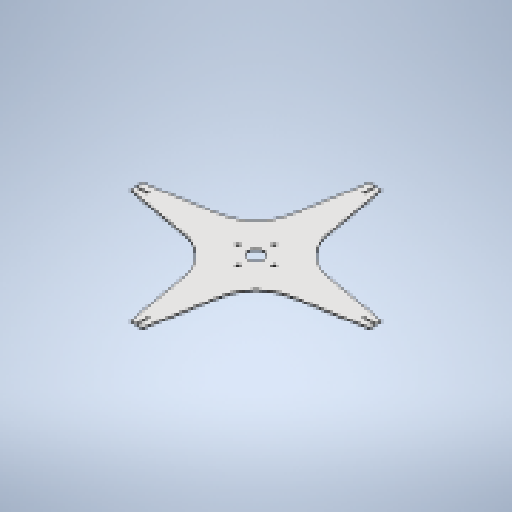
# Autodesk Inventor part: TRM 030 star main
Saved by Autodesk Inventor 2025 (Build 290162010, 162A)
## iProperties
Created: 2024-08-07
Part Number: TRM 030 star main
Material: AISI 304
Document SubType Name: Sheet Metal
Designer: admin
Stock Number: ТРМ 015 левый борт основное
Density: 8.02768 g/cm^3
Flat Pattern Width: 39.95 cm
Flat Pattern Length: 39.95 cm
Flat Pattern Area: 1596 cm^2
Sheet Metal Rule: AISI304 2mm Die16
Sheet Metal Width: 399,500 mm
Sheet Metal Length: 399,500 mm
Sheet Metal Area: 159600,000 mm^2
Appearance: Default
Author: pokla
Autodesk Inventor part; units mm, degrees
ref_plane "YZ Plane" through (0, 0, 0) normal (1, 0, 0) x (0, 1, 0)
ref_plane "XZ Plane" through (0, 0, 0) normal (0, 1, 0) x (-1, 0, 0)
ref_plane "XY Plane" through (0, 0, 0) normal (0, 0, 1) x (1, 0, 0)
sketch "Sketch1" plane through (0, 0, 0) normal (0, 0, 1) x (1, 0, 0)
  circle A0 centre (0, 0) radius 37.5 construction
  circle A1 centre (0, 0) radius 12.5
  line L0 (0, 12.5) -> (35.3553, 12.5) construction
  line L1 (0, -12.5) -> (35.3553, -12.5) construction
  circle A2 centre (0, 0) radius 200
  dimension "d15" = 25
  dimension "d16" = 75
  dimension "d25" = 400
  measures "d15" diameter of A1
  measures "d16" diameter of A0
  measures "d25" diameter of A2
extrude "Plate1" add sketch "Sketch1" along normal blind 2
sketch "Sketch2" plane through (0, 0, 0) normal (0, 0, -1) x (-1, 0, 0)
  line L0 (18.691, -4.6928) -> (218.691, -4.6928) construction
  line L1 (218.691, -4.6928) -> (218.691, -24.6928) construction
  line L2 (218.691, -24.6928) -> (18.691, -24.6928) construction
  line L3 (18.691, -24.6928) -> (18.691, -4.6928) construction
  point P0 (0, 0)
  point P1 (-251, -525)
  dimension "d6" = 200
  dimension "d9" = 20
  constraints: 2 other
  measures "d6" distance of L0.start L0.end
  measures "d9" distance of L0.end L1.end
mark "Mark1"
sketch "Sketch4" plane through (0, 0, 2) normal (0, 0, 1) x (1, 0, 0)
  circle A0 centre (0, 0) radius 12.5 construction
  circle A1 centre (0, 0) radius 200 projected
  line L0 (0, 0) -> (200, 0) construction
  line L1 (0, 0) -> (141.4214, 141.4214) construction
  line L2 (-10, 199.7498) -> (10, 199.7498)
  circle A2 centre (0, 0) radius 200 projected
  line L3 (199.7498, -10) -> (199.7498, 10)
  line L4 (10, 199.7498) -> (29.3236, 90.1605)
  arc A3 (29.3236, 90.1605) -> (90.1605, 29.3236) centre (103.1841, 103.1841) ccw
  line L5 (90.1605, 29.3236) -> (199.7498, 10)
  line L6 (-1.05, 199.7498) -> (-1.05, 179.7498)
  line L7 (-1.05, 179.7498) -> (1.05, 179.7498)
  line L8 (1.05, 179.7498) -> (1.05, 199.7498)
  circle A4 centre (0, 30) radius 3
  line L9 (0, 30) -> (0, 0) construction
  circle A5 centre (0, 0) radius 30 construction
  point P0 (0, 179.7498)
  point P1 (0, 199.7498)
  point P2 (199.7498, 10)
  point P3 (10, 199.7498)
  point P4 (10, 199.7498)
  dimension "d39" = 60
  dimension "d28" = 20
  dimension "d29" = 45
  dimension "d30" = 10
  dimension "d31" = 75
  dimension "d32" = 2.1
  dimension "d33" = 20
  dimension "d40" = 90
  dimension "d41" = 6
  constraints: 20 end point, 8 point on circle, 3 point on line, 2 centre point, 2 equal length, 2 midpoint, 2 perpendicular, 2 tangent, 2 vertical, 2 vertical alignment, 1 coincident, 1 horizontal, 2 other
  measures "d28" distance of L2.start L2.end
  measures "d29" angle of L0 L1
  measures "d30" angle of L0 L5
  measures "d31" radius of A3
  measures "d32" distance of L6.end L7.end
  measures "d33" distance of L6.start L6.end
  measures "d40" angle of L0 L9
  measures "d41" diameter of A4
extrude "Cut2" cut sketch "Sketch4" against normal blind 2 contours L5 A3 L4 A1 | L2 A1 | L8 L7 L6 L2 | A4
pattern_circular "Circular Pattern2" count 4 over 360 about axis through (0, 0, 0) along (0, 0, 1) of "Cut2"
equation "\"JacobiRadiusSize\" = BendRadius"
equation "\"d2\" = Thickness"
equation "\"BendReliefWidth\" = Thickness"
equation "\"BendReliefDepth\" = 0.5 * Thickness"
equation "\"CornerReliefSize\" = 4 * Thickness"
equation "\"MinimumRemnant\" = 2 * Thickness"
equation "\"TransitionRadius\" = BendRadius"
equation "\"GapSize\" = Thickness"
equation "\"BendRadius\" = 2.75"
equation "\"Thickness\" = 2"
body "Solid1"
